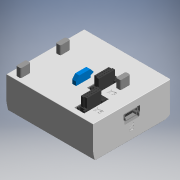
# Autodesk Inventor part: 8070984 CDSB-A1
Saved by Autodesk Inventor 2017.3 (Build 213256000, 256)
## iProperties
Part Number: 8070984 CDSB-A1
Material: Generic
Catalog Web Link: www.cadenas.de
Description: CDSB-Operator unit
Vendor: FESTO
Document SubType Name: Modeling
Designer: partserver
Manufacturer: FESTO
Mass: 36.6 g
Surface Area: 99.6497 cm^2
Volume: 42.8826 cm^3
Density: 1 g/cm^3
Appearance: PSOLRGB-175-175-175
Category: PARTsolutions
Company: FESTO
Title: 8070984 CDSB-A1
Author: Cadenas PARTsolutions
Comments: Operator unit
PSOL_IDENT_0: {$CADENAS_DATA\23d-libs\festo\parts\c\cdsb\cdsb.prj},168 {VTYP=3D},{NB=8070984 CDSB-A1},{LINA=807098
PSOL_IDENT_1: 4 CDSB-A1},{NN=CDSB},{DATE=28.02.2020 14:10:31},{GEOMDATE=22.06.2018 09:50:38},{VERSION=},{LINEID=10
PSOL_IDENT_2: },{WBVAR=},{WBNUMERIC=}  {NB=8070984 CDSB-A1},{LINA=8070984 CDSB-A1},{KT=DUMMY},{TNR=8070984},{TYP=C
PSOL_IDENT_3: DSB-A1},{CNSMASSEXACT=0.0366}
NB: 8070984 CDSB-A1
NN: CDSB
NT: Operator unit
NBSYN: $TNR. $TYP.
LINA: 8070984 CDSB-A1
CATALOG: Festo
TNR: 8070984
TYP: CDSB-A1
CNSMASSEXACT: 0.0366
SUPPLIER: FESTO
ARTICLENO: 8070984 CDSB-A1
BOMINFO: 8070984 CDSB-A1
CREATOR: CADENAS GmbH
Autodesk Inventor part; units mm, degrees
ref_plane "YZ Plane" through (0, 0, 0) normal (1, 0, 0) x (0, 1, 0)
ref_plane "XZ Plane" through (0, 0, 0) normal (0, 1, 0) x (-1, 0, 0)
ref_plane "XY Plane" through (0, 0, 0) normal (0, 0, 1) x (1, 0, 0)
sketch "Sketch_1" plane through (0, 0, 0) normal (1, 0, 0) x (0, 1, 0)
  line L0 (37.9928, 19.588) -> (8.2914, 19.588)
  arc A0 (8.2914, 19.588) -> (1.2796, 18.6197) centre (13.185, -41.717) ccw
  arc A1 (1.2796, 18.6197) -> (1.0492, 18.4076) centre (1.3377, 18.3253) ccw
  arc A2 (1.0492, 18.4076) -> (0, 12.918) centre (31.3426, 9.7728) ccw
  line L1 (0, 12.918) -> (0, 0.2)
  arc A3 (0, 0.2) -> (0.2, 0) centre (0.2, 0.2) ccw
  line L2 (0.2, 0) -> (44.8, 0)
  arc A4 (44.8, 0) -> (45, 0.2) centre (44.8, 0.2) ccw
  line L3 (45, 0.2) -> (45, 17.0653)
  arc A5 (45, 17.0653) -> (44.8438, 17.3286) centre (44.7, 17.0653) ccw
  arc A6 (44.8438, 17.3286) -> (37.9928, 19.588) centre (35.257, -0.224) ccw
  constraints: 14 point on circle, 8 end point, 7 centre point
extrude "Extrusion1" add sketch "Sketch_1" along normal mid plane 50
sketch "Sketch_2" plane through (0, 0, 0) normal (0, 1, 0) x (-1, 0, 0)
  line L0 (30, 25) -> (-30, 25)
  line L1 (-30, 25) -> (-30, -5)
  line L2 (-30, -5) -> (30, -5)
  line L3 (30, -5) -> (30, 25)
  line L4 (25, 0.2) -> (25, 18.5987)
  arc A0 (25, 18.5987) -> (24.7656, 18.8915) centre (24.7, 18.5987) ccw
  arc A1 (24.7656, 18.8915) -> (20, 19.588) centre (17.7679, -12.3341) ccw
  line L5 (20, 19.588) -> (-20, 19.588)
  arc A2 (-20, 19.588) -> (-24.7656, 18.8915) centre (-17.7679, -12.3341) ccw
  arc A3 (-24.7656, 18.8915) -> (-25, 18.5987) centre (-24.7, 18.5987) ccw
  line L6 (-25, 18.5987) -> (-25, 0.2)
  arc A4 (-25, 0.2) -> (-24.8, 0) centre (-24.8, 0.2) ccw
  line L7 (-24.8, 0) -> (24.8, 0)
  arc A5 (24.8, 0) -> (25, 0.2) centre (24.8, 0.2) ccw
  constraints: 16 end point, 12 point on circle, 6 centre point
extrude "Extrusion2" cut sketch "Sketch_2" along normal blind 50
sketch "Sketch_3" plane through (0, 0, 0) normal (0, 0, 1) x (1, 0, 0)
  line L0 (-30, 35) -> (-25, 35)
  line L1 (-25, 35) -> (-25, 44.2)
  arc A0 (-24.2, 45) -> (-25, 44.2) centre (-24.2, 44.2) ccw
  line L2 (-24.2, 45) -> (24.2, 45)
  arc A1 (25, 44.2) -> (24.2, 45) centre (24.2, 44.2) ccw
  line L3 (25, 44.2) -> (25, 35)
  line L4 (25, 35) -> (30, 35)
  line L5 (30, 35) -> (30, 50)
  line L6 (30, 50) -> (-30, 50)
  line L7 (-30, 50) -> (-30, 35)
  constraints: 16 end point, 4 point on circle, 2 centre point
extrude "Extrusion3" cut sketch "Sketch_3" along normal blind 20
sketch "Sketch_4" plane through (0, 0, 0) normal (1, 0, 0) x (0, 1, 0)
  line L0 (45.89, 10.51) -> (45, 10.51)
  line L1 (45, 10.51) -> (45, 2.16)
  line L2 (45, 2.16) -> (45.89, 2.16)
  arc A0 (45.89, 2.16) -> (46.69, 2.96) centre (45.89, 2.96) ccw
  line L3 (46.69, 2.96) -> (46.69, 9.71)
  arc A1 (46.69, 9.71) -> (45.89, 10.51) centre (45.89, 9.71) ccw
  constraints: 8 end point, 4 point on circle, 2 centre point
extrude "Extrusion4" add sketch "Sketch_4" along normal mid plane 21.6
sketch "Sketch_5" plane through (0, 0, 0) normal (0, 0, 1) x (1, 0, 0)
  line L0 (-12.8, 48.69) -> (-12.8, 45)
  line L1 (-12.8, 45) -> (-10.8, 45)
  line L2 (-10.8, 45) -> (-10.8, 46.14)
  arc A0 (-10.25, 46.69) -> (-10.8, 46.14) centre (-10.25, 46.14) ccw
  line L3 (-10.25, 46.69) -> (10.25, 46.69)
  arc A1 (10.8, 46.14) -> (10.25, 46.69) centre (10.25, 46.14) ccw
  line L4 (10.8, 46.14) -> (10.8, 45)
  line L5 (10.8, 45) -> (12.8, 45)
  line L6 (12.8, 45) -> (12.8, 48.69)
  line L7 (12.8, 48.69) -> (-12.8, 48.69)
  constraints: 16 end point, 4 point on circle, 2 centre point
extrude "Extrusion5" cut sketch "Sketch_5" along normal blind 15
sketch "Sketch_6" plane through (0, 0, 0) normal (1, 0, 0) x (0, 1, 0)
  line L0 (22.64, 0) -> (14.2, 0)
  line L1 (14.2, 0) -> (14.2, -2.17)
  line L2 (14.2, -2.17) -> (15.9896, -4.38)
  line L3 (15.9896, -4.38) -> (22.1436, -4.38)
  arc A0 (22.1436, -4.38) -> (22.5649, -4.1835) centre (22.1436, -3.83) ccw
  line L4 (22.5649, -4.1835) -> (24.33, -2.08)
  line L5 (24.33, -2.08) -> (24.33, -1.9851)
  line L6 (24.33, -1.9851) -> (22.64, -1.3364)
  line L7 (22.64, -1.3364) -> (22.64, 0)
  constraints: 16 end point, 2 point on circle, 1 centre point
extrude "Extrusion6" add sketch "Sketch_6" along normal mid plane 2.3
sketch "Sketch_7" plane through (0, 0, 0) normal (0, 0, 1) x (1, 0, 0)
  line L0 (-10.837, 30.43) -> (-10.837, 16.63)
  arc A0 (-10.837, 16.63) -> (-10.637, 16.43) centre (-10.637, 16.63) ccw
  line L1 (-10.637, 16.43) -> (-5.337, 16.43)
  arc A1 (-5.337, 16.43) -> (-5.137, 16.63) centre (-5.337, 16.63) ccw
  line L2 (-5.137, 16.63) -> (-5.137, 30.43)
  arc A2 (-5.137, 30.43) -> (-5.337, 30.63) centre (-5.337, 30.43) ccw
  line L3 (-5.337, 30.63) -> (-10.637, 30.63)
  arc A3 (-10.637, 30.63) -> (-10.837, 30.43) centre (-10.637, 30.43) ccw
  constraints: 8 end point, 8 point on circle, 4 centre point
extrude "Extrusion7" cut sketch "Sketch_7" along normal blind 4.5
sketch "Sketch_8" plane through (0, 0, 0) normal (0, 0, 1) x (1, 0, 0)
  line L0 (-17.136, 16.87) -> (-17.136, 3.07)
  arc A0 (-17.136, 3.07) -> (-16.936, 2.87) centre (-16.936, 3.07) ccw
  line L1 (-16.936, 2.87) -> (-11.636, 2.87)
  arc A1 (-11.636, 2.87) -> (-11.436, 3.07) centre (-11.636, 3.07) ccw
  line L2 (-11.436, 3.07) -> (-11.436, 16.87)
  arc A2 (-11.436, 16.87) -> (-11.636, 17.07) centre (-11.636, 16.87) ccw
  line L3 (-11.636, 17.07) -> (-16.936, 17.07)
  arc A3 (-16.936, 17.07) -> (-17.136, 16.87) centre (-16.936, 16.87) ccw
  constraints: 8 end point, 8 point on circle, 4 centre point
extrude "Extrusion8" cut sketch "Sketch_8" along normal blind 4.5
sketch "Sketch_9" plane through (0, 0, -0.15) normal (0, 0, 1) x (1, 0, 0)
  line L0 (-10.055, 19.535) -> (-10.055, 17.22)
  line L1 (-10.055, 17.22) -> (-9.255, 17.22)
  line L2 (-9.255, 17.22) -> (-9.255, 18.385)
  line L3 (-9.255, 18.385) -> (-6.655, 18.385)
  line L4 (-6.655, 18.385) -> (-6.655, 17.22)
  line L5 (-6.655, 17.22) -> (-5.855, 17.22)
  line L6 (-5.855, 17.22) -> (-5.855, 19.535)
  line L7 (-5.855, 19.535) -> (-6.43, 19.535)
  line L8 (-6.43, 19.535) -> (-6.43, 27.605)
  line L9 (-6.43, 27.605) -> (-5.855, 27.605)
  line L10 (-5.855, 27.605) -> (-5.855, 29.92)
  line L11 (-5.855, 29.92) -> (-6.655, 29.92)
  line L12 (-6.655, 29.92) -> (-6.655, 28.755)
  line L13 (-6.655, 28.755) -> (-9.255, 28.755)
  line L14 (-9.255, 28.755) -> (-9.255, 29.92)
  line L15 (-9.255, 29.92) -> (-10.055, 29.92)
  line L16 (-10.055, 29.92) -> (-10.055, 27.605)
  line L17 (-10.055, 27.605) -> (-9.48, 27.605)
  line L18 (-9.48, 27.605) -> (-9.48, 19.535)
  line L19 (-9.48, 19.535) -> (-10.055, 19.535)
  constraints: 40 end point
extrude "Extrusion9" add sketch "Sketch_9" along normal blind 4.65
sketch "Sketch_10" plane through (0, 0, -0.15) normal (0, 0, 1) x (1, 0, 0)
  line L0 (-16.35, 5.975) -> (-16.35, 3.66)
  line L1 (-16.35, 3.66) -> (-15.55, 3.66)
  line L2 (-15.55, 3.66) -> (-15.55, 4.825)
  line L3 (-15.55, 4.825) -> (-12.95, 4.825)
  line L4 (-12.95, 4.825) -> (-12.95, 3.66)
  line L5 (-12.95, 3.66) -> (-12.15, 3.66)
  line L6 (-12.15, 3.66) -> (-12.15, 5.975)
  line L7 (-12.15, 5.975) -> (-12.725, 5.975)
  line L8 (-12.725, 5.975) -> (-12.725, 14.045)
  line L9 (-12.725, 14.045) -> (-12.15, 14.045)
  line L10 (-12.15, 14.045) -> (-12.15, 16.36)
  line L11 (-12.15, 16.36) -> (-12.95, 16.36)
  line L12 (-12.95, 16.36) -> (-12.95, 15.195)
  line L13 (-12.95, 15.195) -> (-15.55, 15.195)
  line L14 (-15.55, 15.195) -> (-15.55, 16.36)
  line L15 (-15.55, 16.36) -> (-16.35, 16.36)
  line L16 (-16.35, 16.36) -> (-16.35, 14.045)
  line L17 (-16.35, 14.045) -> (-15.775, 14.045)
  line L18 (-15.775, 14.045) -> (-15.775, 5.975)
  line L19 (-15.775, 5.975) -> (-16.35, 5.975)
  constraints: 40 end point
extrude "Extrusion10" add sketch "Sketch_10" along normal blind 4.65
sketch "Sketch_11" plane through (0, 0, -5.35) normal (0, 0, 1) x (1, 0, 0)
  line L0 (-9.48, 18.96) -> (-7.93, 18.96)
  line L1 (-7.93, 18.96) -> (-7.93, 19.46)
  line L2 (-7.93, 19.46) -> (-6.43, 19.46)
  line L3 (-6.43, 19.46) -> (-6.43, 27.83)
  line L4 (-6.43, 27.83) -> (-7.93, 27.83)
  line L5 (-7.93, 27.83) -> (-7.93, 28.33)
  line L6 (-7.93, 28.33) -> (-9.48, 28.33)
  line L7 (-9.48, 28.33) -> (-9.48, 18.96)
  constraints: 16 end point
extrude "Extrusion11" add sketch "Sketch_11" along normal blind 5.2
sketch "Sketch_12" plane through (0, 0, -5.35) normal (0, 0, 1) x (1, 0, 0)
  line L0 (-15.775, 5.83) -> (-14.275, 5.83)
  line L1 (-14.275, 5.83) -> (-14.275, 5.33)
  line L2 (-14.275, 5.33) -> (-12.725, 5.33)
  line L3 (-12.725, 5.33) -> (-12.725, 14.7)
  line L4 (-12.725, 14.7) -> (-14.275, 14.7)
  line L5 (-14.275, 14.7) -> (-14.275, 14.2)
  line L6 (-14.275, 14.2) -> (-15.775, 14.2)
  line L7 (-15.775, 14.2) -> (-15.775, 5.83)
  constraints: 16 end point
extrude "Extrusion12" add sketch "Sketch_12" along normal blind 5.2
sketch "Sketch_13" plane through (0, 0, -5.35) normal (0, 0, 1) x (1, 0, 0)
  line L0 (-8.7, 26.53) -> (-8.3, 26.53)
  line L1 (-8.3, 26.53) -> (-8.3, 27.13)
  line L2 (-8.3, 27.13) -> (-8.7, 27.13)
  line L3 (-8.7, 27.13) -> (-8.7, 26.53)
  constraints: 8 end point
extrude "Extrusion13" cut sketch "Sketch_13" along normal blind 0.5
sketch "Pattern_1_SKETCH_1" plane through (0, 0, -5.35) normal (0, 0, 1) x (1, 0, 0)
  line L0 (-7.43, 26.53) -> (-7.03, 26.53)
  line L1 (-7.03, 26.53) -> (-7.03, 27.13)
  line L2 (-7.03, 27.13) -> (-7.43, 27.13)
  line L3 (-7.43, 27.13) -> (-7.43, 26.53)
  constraints: 8 end point
sketch "Pattern_1_SKETCH_2" plane through (0, 0, -5.35) normal (0, 0, 1) x (1, 0, 0)
  line L0 (-7.43, 25.26) -> (-7.03, 25.26)
  line L1 (-7.03, 25.26) -> (-7.03, 25.86)
  line L2 (-7.03, 25.86) -> (-7.43, 25.86)
  line L3 (-7.43, 25.86) -> (-7.43, 25.26)
  constraints: 8 end point
sketch "Pattern_1_SKETCH_3" plane through (0, 0, -5.35) normal (0, 0, 1) x (1, 0, 0)
  line L0 (-7.43, 23.99) -> (-7.03, 23.99)
  line L1 (-7.03, 23.99) -> (-7.03, 24.59)
  line L2 (-7.03, 24.59) -> (-7.43, 24.59)
  line L3 (-7.43, 24.59) -> (-7.43, 23.99)
  constraints: 8 end point
sketch "Pattern_1_SKETCH_4" plane through (0, 0, -5.35) normal (0, 0, 1) x (1, 0, 0)
  line L0 (-7.43, 22.72) -> (-7.03, 22.72)
  line L1 (-7.03, 22.72) -> (-7.03, 23.32)
  line L2 (-7.03, 23.32) -> (-7.43, 23.32)
  line L3 (-7.43, 23.32) -> (-7.43, 22.72)
  constraints: 8 end point
sketch "Pattern_1_SKETCH_5" plane through (0, 0, -5.35) normal (0, 0, 1) x (1, 0, 0)
  line L0 (-7.43, 21.45) -> (-7.03, 21.45)
  line L1 (-7.03, 21.45) -> (-7.03, 22.05)
  line L2 (-7.03, 22.05) -> (-7.43, 22.05)
  line L3 (-7.43, 22.05) -> (-7.43, 21.45)
  constraints: 8 end point
sketch "Pattern_1_SKETCH_6" plane through (0, 0, -5.35) normal (0, 0, 1) x (1, 0, 0)
  line L0 (-7.43, 20.18) -> (-7.03, 20.18)
  line L1 (-7.03, 20.18) -> (-7.03, 20.78)
  line L2 (-7.03, 20.78) -> (-7.43, 20.78)
  line L3 (-7.43, 20.78) -> (-7.43, 20.18)
  constraints: 8 end point
sketch "Pattern_1_SKETCH_7" plane through (0, 0, -5.35) normal (0, 0, 1) x (1, 0, 0)
  line L0 (-8.7, 25.26) -> (-8.3, 25.26)
  line L1 (-8.3, 25.26) -> (-8.3, 25.86)
  line L2 (-8.3, 25.86) -> (-8.7, 25.86)
  line L3 (-8.7, 25.86) -> (-8.7, 25.26)
  constraints: 8 end point
sketch "Pattern_1_SKETCH_8" plane through (0, 0, -5.35) normal (0, 0, 1) x (1, 0, 0)
  line L0 (-8.7, 23.99) -> (-8.3, 23.99)
  line L1 (-8.3, 23.99) -> (-8.3, 24.59)
  line L2 (-8.3, 24.59) -> (-8.7, 24.59)
  line L3 (-8.7, 24.59) -> (-8.7, 23.99)
  constraints: 8 end point
sketch "Pattern_1_SKETCH_9" plane through (0, 0, -5.35) normal (0, 0, 1) x (1, 0, 0)
  line L0 (-8.7, 22.72) -> (-8.3, 22.72)
  line L1 (-8.3, 22.72) -> (-8.3, 23.32)
  line L2 (-8.3, 23.32) -> (-8.7, 23.32)
  line L3 (-8.7, 23.32) -> (-8.7, 22.72)
  constraints: 8 end point
sketch "Pattern_1_SKETCH_10" plane through (0, 0, -5.35) normal (0, 0, 1) x (1, 0, 0)
  line L0 (-8.7, 21.45) -> (-8.3, 21.45)
  line L1 (-8.3, 21.45) -> (-8.3, 22.05)
  line L2 (-8.3, 22.05) -> (-8.7, 22.05)
  line L3 (-8.7, 22.05) -> (-8.7, 21.45)
  constraints: 8 end point
sketch "Pattern_1_SKETCH_11" plane through (0, 0, -5.35) normal (0, 0, 1) x (1, 0, 0)
  line L0 (-8.7, 20.18) -> (-8.3, 20.18)
  line L1 (-8.3, 20.18) -> (-8.3, 20.78)
  line L2 (-8.3, 20.78) -> (-8.7, 20.78)
  line L3 (-8.7, 20.78) -> (-8.7, 20.18)
  constraints: 8 end point
sketch "Pattern_1_SKETCH_12" plane through (0, 0, -5.35) normal (0, 0, 1) x (1, 0, 0)
  line L0 (-15, 12.97) -> (-14.6, 12.97)
  line L1 (-14.6, 12.97) -> (-14.6, 13.57)
  line L2 (-14.6, 13.57) -> (-15, 13.57)
  line L3 (-15, 13.57) -> (-15, 12.97)
  constraints: 8 end point
sketch "Pattern_1_SKETCH_13" plane through (0, 0, -5.35) normal (0, 0, 1) x (1, 0, 0)
  line L0 (-13.73, 12.97) -> (-13.33, 12.97)
  line L1 (-13.33, 12.97) -> (-13.33, 13.57)
  line L2 (-13.33, 13.57) -> (-13.73, 13.57)
  line L3 (-13.73, 13.57) -> (-13.73, 12.97)
  constraints: 8 end point
sketch "Pattern_1_SKETCH_14" plane through (0, 0, -5.35) normal (0, 0, 1) x (1, 0, 0)
  line L0 (-15, 11.7) -> (-14.6, 11.7)
  line L1 (-14.6, 11.7) -> (-14.6, 12.3)
  line L2 (-14.6, 12.3) -> (-15, 12.3)
  line L3 (-15, 12.3) -> (-15, 11.7)
  constraints: 8 end point
sketch "Pattern_1_SKETCH_15" plane through (0, 0, -5.35) normal (0, 0, 1) x (1, 0, 0)
  line L0 (-13.73, 11.7) -> (-13.33, 11.7)
  line L1 (-13.33, 11.7) -> (-13.33, 12.3)
  line L2 (-13.33, 12.3) -> (-13.73, 12.3)
  line L3 (-13.73, 12.3) -> (-13.73, 11.7)
  constraints: 8 end point
sketch "Pattern_1_SKETCH_16" plane through (0, 0, -5.35) normal (0, 0, 1) x (1, 0, 0)
  line L0 (-15, 10.43) -> (-14.6, 10.43)
  line L1 (-14.6, 10.43) -> (-14.6, 11.03)
  line L2 (-14.6, 11.03) -> (-15, 11.03)
  line L3 (-15, 11.03) -> (-15, 10.43)
  constraints: 8 end point
sketch "Pattern_1_SKETCH_17" plane through (0, 0, -5.35) normal (0, 0, 1) x (1, 0, 0)
  line L0 (-13.73, 10.43) -> (-13.33, 10.43)
  line L1 (-13.33, 10.43) -> (-13.33, 11.03)
  line L2 (-13.33, 11.03) -> (-13.73, 11.03)
  line L3 (-13.73, 11.03) -> (-13.73, 10.43)
  constraints: 8 end point
sketch "Pattern_1_SKETCH_18" plane through (0, 0, -5.35) normal (0, 0, 1) x (1, 0, 0)
  line L0 (-15, 9.16) -> (-14.6, 9.16)
  line L1 (-14.6, 9.16) -> (-14.6, 9.76)
  line L2 (-14.6, 9.76) -> (-15, 9.76)
  line L3 (-15, 9.76) -> (-15, 9.16)
  constraints: 8 end point
sketch "Pattern_1_SKETCH_19" plane through (0, 0, -5.35) normal (0, 0, 1) x (1, 0, 0)
  line L0 (-13.73, 9.16) -> (-13.33, 9.16)
  line L1 (-13.33, 9.16) -> (-13.33, 9.76)
  line L2 (-13.33, 9.76) -> (-13.73, 9.76)
  line L3 (-13.73, 9.76) -> (-13.73, 9.16)
  constraints: 8 end point
sketch "Pattern_1_SKETCH_20" plane through (0, 0, -5.35) normal (0, 0, 1) x (1, 0, 0)
  line L0 (-15, 7.89) -> (-14.6, 7.89)
  line L1 (-14.6, 7.89) -> (-14.6, 8.49)
  line L2 (-14.6, 8.49) -> (-15, 8.49)
  line L3 (-15, 8.49) -> (-15, 7.89)
  constraints: 8 end point
sketch "Pattern_1_SKETCH_21" plane through (0, 0, -5.35) normal (0, 0, 1) x (1, 0, 0)
  line L0 (-13.73, 7.89) -> (-13.33, 7.89)
  line L1 (-13.33, 7.89) -> (-13.33, 8.49)
  line L2 (-13.33, 8.49) -> (-13.73, 8.49)
  line L3 (-13.73, 8.49) -> (-13.73, 7.89)
  constraints: 8 end point
sketch "Pattern_1_SKETCH_22" plane through (0, 0, -5.35) normal (0, 0, 1) x (1, 0, 0)
  line L0 (-15, 6.62) -> (-14.6, 6.62)
  line L1 (-14.6, 6.62) -> (-14.6, 7.22)
  line L2 (-14.6, 7.22) -> (-15, 7.22)
  line L3 (-15, 7.22) -> (-15, 6.62)
  constraints: 8 end point
sketch "Pattern_1_SKETCH_23" plane through (0, 0, -5.35) normal (0, 0, 1) x (1, 0, 0)
  line L0 (-13.73, 6.62) -> (-13.33, 6.62)
  line L1 (-13.33, 6.62) -> (-13.33, 7.22)
  line L2 (-13.33, 7.22) -> (-13.73, 7.22)
  line L3 (-13.73, 7.22) -> (-13.73, 6.62)
  constraints: 8 end point
extrude "Extrusion14" cut sketch "Pattern_1_SKETCH_1" along normal blind 0.5
extrude "Extrusion15" cut sketch "Pattern_1_SKETCH_2" along normal blind 0.5
extrude "Extrusion16" cut sketch "Pattern_1_SKETCH_3" along normal blind 0.5
extrude "Extrusion17" cut sketch "Pattern_1_SKETCH_4" along normal blind 0.5
extrude "Extrusion18" cut sketch "Pattern_1_SKETCH_5" along normal blind 0.5
extrude "Extrusion19" cut sketch "Pattern_1_SKETCH_6" along normal blind 0.5
extrude "Extrusion20" cut sketch "Pattern_1_SKETCH_7" along normal blind 0.5
extrude "Extrusion21" cut sketch "Pattern_1_SKETCH_8" along normal blind 0.5
extrude "Extrusion22" cut sketch "Pattern_1_SKETCH_9" along normal blind 0.5
extrude "Extrusion23" cut sketch "Pattern_1_SKETCH_10" along normal blind 0.5
extrude "Extrusion24" cut sketch "Pattern_1_SKETCH_11" along normal blind 0.5
extrude "Extrusion25" cut sketch "Pattern_1_SKETCH_12" along normal blind 0.5
extrude "Extrusion26" cut sketch "Pattern_1_SKETCH_13" along normal blind 0.5
extrude "Extrusion27" cut sketch "Pattern_1_SKETCH_14" along normal blind 0.5
extrude "Extrusion28" cut sketch "Pattern_1_SKETCH_15" along normal blind 0.5
extrude "Extrusion29" cut sketch "Pattern_1_SKETCH_16" along normal blind 0.5
extrude "Extrusion30" cut sketch "Pattern_1_SKETCH_17" along normal blind 0.5
extrude "Extrusion31" cut sketch "Pattern_1_SKETCH_18" along normal blind 0.5
extrude "Extrusion32" cut sketch "Pattern_1_SKETCH_19" along normal blind 0.5
extrude "Extrusion33" cut sketch "Pattern_1_SKETCH_20" along normal blind 0.5
extrude "Extrusion34" cut sketch "Pattern_1_SKETCH_21" along normal blind 0.5
extrude "Extrusion35" cut sketch "Pattern_1_SKETCH_22" along normal blind 0.5
extrude "Extrusion36" cut sketch "Pattern_1_SKETCH_23" along normal blind 0.5
sketch "Sketch_15" plane through (0, 0, 0) normal (0, 0, 1) x (1, 0, 0)
  arc A0 (18.65, 25.55) -> (19.35, 24.85) centre (19.35, 25.55) ccw
  line L0 (19.35, 24.85) -> (20.7, 24.85)
  arc A1 (20.7, 24.85) -> (21.4, 25.55) centre (20.7, 25.55) ccw
  line L1 (21.4, 25.55) -> (21.4, 29.9)
  arc A2 (21.4, 29.9) -> (20.7, 30.6) centre (20.7, 29.9) ccw
  line L2 (20.7, 30.6) -> (19.35, 30.6)
  arc A3 (19.35, 30.6) -> (18.65, 29.9) centre (19.35, 29.9) ccw
  line L3 (18.65, 29.9) -> (18.65, 25.55)
  constraints: 8 end point, 8 point on circle, 4 centre point
extrude "Extrusion37" add sketch "Sketch_15" against normal blind 5
sketch "Sketch_16" plane through (0, 0, 0) normal (0, 0, 1) x (1, 0, 0)
  arc A0 (18.65, 2.7) -> (19.35, 2) centre (19.35, 2.7) ccw
  line L0 (19.35, 2) -> (20.7, 2)
  arc A1 (20.7, 2) -> (21.4, 2.7) centre (20.7, 2.7) ccw
  line L1 (21.4, 2.7) -> (21.4, 7.05)
  arc A2 (21.4, 7.05) -> (20.7, 7.75) centre (20.7, 7.05) ccw
  line L2 (20.7, 7.75) -> (19.35, 7.75)
  arc A3 (19.35, 7.75) -> (18.65, 7.05) centre (19.35, 7.05) ccw
  line L3 (18.65, 7.05) -> (18.65, 2.7)
  constraints: 8 end point, 8 point on circle, 4 centre point
extrude "Extrusion38" add sketch "Sketch_16" against normal blind 5
sketch "Sketch_17" plane through (0, 0, 0) normal (0, 0, 1) x (1, 0, 0)
  arc A0 (-16.1, 25.55) -> (-15.4, 24.85) centre (-15.4, 25.55) ccw
  line L0 (-15.4, 24.85) -> (-14.05, 24.85)
  arc A1 (-14.05, 24.85) -> (-13.35, 25.55) centre (-14.05, 25.55) ccw
  line L1 (-13.35, 25.55) -> (-13.35, 29.9)
  arc A2 (-13.35, 29.9) -> (-14.05, 30.6) centre (-14.05, 29.9) ccw
  line L2 (-14.05, 30.6) -> (-15.4, 30.6)
  arc A3 (-15.4, 30.6) -> (-16.1, 29.9) centre (-15.4, 29.9) ccw
  line L3 (-16.1, 29.9) -> (-16.1, 25.55)
  constraints: 8 end point, 8 point on circle, 4 centre point
extrude "Extrusion39" add sketch "Sketch_17" against normal blind 5
sketch "Sketch_18" plane through (-18.6, 0, 0) normal (1, 0, 0) x (0, 0, -1)
  line L0 (-9.6, 26.25) -> (-9.6, 18.75)
  arc A0 (-9.6, 18.75) -> (-9.1, 18.25) centre (-9.1, 18.75) ccw
  line L1 (-9.1, 18.25) -> (-8.1203, 18.25)
  arc A1 (-7.8972, 18.1975) -> (-8.1203, 18.25) centre (-8.1203, 17.75) ccw
  line L2 (-7.8972, 18.1975) -> (-7.1051, 17.8025)
  arc A2 (-7.1051, 17.8025) -> (-6.882, 17.75) centre (-6.882, 18.25) ccw
  line L3 (-6.882, 17.75) -> (-4.5, 17.75)
  arc A3 (-4.5, 17.75) -> (-4, 18.25) centre (-4.5, 18.25) ccw
  line L4 (-4, 18.25) -> (-4, 26.75)
  arc A4 (-4, 26.75) -> (-4.5, 27.25) centre (-4.5, 26.75) ccw
  line L5 (-4.5, 27.25) -> (-6.882, 27.25)
  arc A5 (-6.882, 27.25) -> (-7.1051, 27.1975) centre (-6.882, 26.75) ccw
  line L6 (-7.1051, 27.1975) -> (-7.8972, 26.8025)
  arc A6 (-8.1203, 26.75) -> (-7.8972, 26.8025) centre (-8.1203, 27.25) ccw
  line L7 (-8.1203, 26.75) -> (-9.1, 26.75)
  arc A7 (-9.1, 26.75) -> (-9.6, 26.25) centre (-9.1, 26.25) ccw
  constraints: 16 end point, 16 point on circle, 8 centre point
extrude "Extrusion40" cut sketch "Sketch_18" against normal blind 6.5
sketch "Sketch_19" plane through (-18.6, 0, 0) normal (1, 0, 0) x (0, 0, -1)
  line L0 (-8.6, 25.335) -> (-8.6, 19.665)
  arc A0 (-8.6, 19.665) -> (-8.1, 19.165) centre (-8.1, 19.665) ccw
  line L1 (-8.1, 19.165) -> (-7.354, 19.165)
  arc A1 (-7.2986, 19.1482) -> (-7.354, 19.165) centre (-7.354, 19.065) ccw
  line L2 (-7.2986, 19.1482) -> (-6.6775, 18.734)
  arc A2 (-6.6775, 18.734) -> (-6.4001, 18.65) centre (-6.4001, 19.15) ccw
  line L3 (-6.4001, 18.65) -> (-5.2, 18.65)
  arc A3 (-5.2, 18.65) -> (-4.7, 19.15) centre (-5.2, 19.15) ccw
  line L4 (-4.7, 19.15) -> (-4.7, 25.85)
  arc A4 (-4.7, 25.85) -> (-5.2, 26.35) centre (-5.2, 25.85) ccw
  line L5 (-5.2, 26.35) -> (-6.4001, 26.35)
  arc A5 (-6.4001, 26.35) -> (-6.6775, 26.266) centre (-6.4001, 25.85) ccw
  line L6 (-6.6775, 26.266) -> (-7.2986, 25.8518)
  arc A6 (-7.354, 25.835) -> (-7.2986, 25.8518) centre (-7.354, 25.935) ccw
  line L7 (-7.354, 25.835) -> (-8.1, 25.835)
  arc A7 (-8.1, 25.835) -> (-8.6, 25.335) centre (-8.1, 25.335) ccw
  line L8 (-8.2, 25.335) -> (-8.2, 19.665)
  arc A8 (-8.2, 19.665) -> (-8.1, 19.565) centre (-8.1, 19.665) ccw
  line L9 (-8.1, 19.565) -> (-7.354, 19.565)
  arc A9 (-7.0766, 19.481) -> (-7.354, 19.565) centre (-7.354, 19.065) ccw
  line L10 (-7.0766, 19.481) -> (-6.4556, 19.0668)
  arc A10 (-6.4556, 19.0668) -> (-6.4001, 19.05) centre (-6.4001, 19.15) ccw
  line L11 (-6.4001, 19.05) -> (-5.2, 19.05)
  arc A11 (-5.2, 19.05) -> (-5.1, 19.15) centre (-5.2, 19.15) ccw
  line L12 (-5.1, 19.15) -> (-5.1, 25.85)
  arc A12 (-5.1, 25.85) -> (-5.2, 25.95) centre (-5.2, 25.85) ccw
  line L13 (-5.2, 25.95) -> (-6.4001, 25.95)
  arc A13 (-6.4001, 25.95) -> (-6.4556, 25.9332) centre (-6.4001, 25.85) ccw
  line L14 (-6.4556, 25.9332) -> (-7.0766, 25.519)
  arc A14 (-7.354, 25.435) -> (-7.0766, 25.519) centre (-7.354, 25.935) ccw
  line L15 (-7.354, 25.435) -> (-8.1, 25.435)
  arc A15 (-8.1, 25.435) -> (-8.2, 25.335) centre (-8.1, 25.335) ccw
  constraints: 32 end point, 32 point on circle, 16 centre point
extrude "Extrusion41" add sketch "Sketch_19" against normal blind 5.9
sketch "Sketch_20" plane through (-18.6, 0, 0) normal (1, 0, 0) x (0, 0, -1)
  arc A0 (-7.63, 20.5388) -> (-7.5609, 20.4437) centre (-7.53, 20.5388) ccw
  line L0 (-7.5609, 20.4437) -> (-6.8874, 20.2249)
  arc A1 (-6.8874, 20.2249) -> (-6.8565, 20.22) centre (-6.8565, 20.32) ccw
  line L1 (-6.8565, 20.22) -> (-6.15, 20.22)
  arc A2 (-6.15, 20.22) -> (-6.05, 20.32) centre (-6.15, 20.32) ccw
  line L2 (-6.05, 20.32) -> (-6.05, 24.67)
  arc A3 (-6.05, 24.67) -> (-6.15, 24.77) centre (-6.15, 24.67) ccw
  line L3 (-6.15, 24.77) -> (-6.8565, 24.77)
  arc A4 (-6.8565, 24.77) -> (-6.8874, 24.7651) centre (-6.8565, 24.67) ccw
  line L4 (-6.8874, 24.7651) -> (-7.5609, 24.5463)
  arc A5 (-7.5609, 24.5463) -> (-7.63, 24.4512) centre (-7.53, 24.4512) ccw
  line L5 (-7.63, 24.4512) -> (-7.63, 20.5388)
  line L6 (-6.87, 23.895) -> (-6.3, 23.895)
  line L7 (-6.3, 23.895) -> (-6.3, 24.295)
  line L8 (-6.3, 24.295) -> (-6.87, 24.295)
  line L9 (-6.87, 24.295) -> (-6.87, 23.895)
  line L10 (-6.87, 23.095) -> (-6.3, 23.095)
  line L11 (-6.3, 23.095) -> (-6.3, 23.495)
  line L12 (-6.3, 23.495) -> (-6.87, 23.495)
  line L13 (-6.87, 23.495) -> (-6.87, 23.095)
  line L14 (-6.87, 22.295) -> (-6.3, 22.295)
  line L15 (-6.3, 22.295) -> (-6.3, 22.695)
  line L16 (-6.3, 22.695) -> (-6.87, 22.695)
  line L17 (-6.87, 22.695) -> (-6.87, 22.295)
  line L18 (-6.87, 21.495) -> (-6.3, 21.495)
  line L19 (-6.3, 21.495) -> (-6.3, 21.895)
  line L20 (-6.3, 21.895) -> (-6.87, 21.895)
  line L21 (-6.87, 21.895) -> (-6.87, 21.495)
  line L22 (-6.87, 20.695) -> (-6.3, 20.695)
  line L23 (-6.3, 20.695) -> (-6.3, 21.095)
  line L24 (-6.3, 21.095) -> (-6.87, 21.095)
  line L25 (-6.87, 21.095) -> (-6.87, 20.695)
  constraints: 52 end point, 12 point on circle, 6 centre point
extrude "Extrusion42" add sketch "Sketch_20" against normal blind 4.55
sketch "Sketch_21" plane through (0, 0, 19.588) normal (0, 0, 1) x (1, 0, 0)
  line L0 (-20.5, 36.85) -> (-20.5, 8.85)
  arc A0 (-20.5, 8.85) -> (-19.5, 7.85) centre (-19.5, 8.85) ccw
  line L1 (-19.5, 7.85) -> (19.5, 7.85)
  arc A1 (19.5, 7.85) -> (20.5, 8.85) centre (19.5, 8.85) ccw
  line L2 (20.5, 8.85) -> (20.5, 36.85)
  arc A2 (20.5, 36.85) -> (19.5, 37.85) centre (19.5, 36.85) ccw
  line L3 (19.5, 37.85) -> (-19.5, 37.85)
  arc A3 (-19.5, 37.85) -> (-20.5, 36.85) centre (-19.5, 36.85) ccw
  constraints: 8 end point, 8 point on circle, 4 centre point
extrude "Extrusion43" cut sketch "Sketch_21" against normal blind 0.6
sketch "Sketch_28" plane through (0, 0, 18.988) normal (0, 0, 1) x (1, 0, 0)
  line L0 (-20.5, 36.85) -> (-20.5, 8.85)
  arc A0 (-20.5, 8.85) -> (-19.5, 7.85) centre (-19.5, 8.85) ccw
  line L1 (-19.5, 7.85) -> (-15.5, 7.85)
  line L2 (-15.5, 7.85) -> (-15.5, 37.85)
  line L3 (-15.5, 37.85) -> (-19.5, 37.85)
  arc A1 (-19.5, 37.85) -> (-20.5, 36.85) centre (-19.5, 36.85) ccw
  constraints: 8 end point, 4 point on circle, 2 centre point
extrude "Extrusion44" add sketch "Sketch_28" along normal blind 0.4
sketch "Sketch_22" plane through (-25, 0, 0) normal (1, 0, 0) x (0, 0, -1)
  line L0 (-13.0625, 21.25) -> (-12.6562, 21.25)
  line L1 (-12.6562, 21.25) -> (-12, 22.2188)
  line L2 (-12, 22.2188) -> (-11.3438, 21.25)
  line L3 (-11.3438, 21.25) -> (-10.9375, 21.25)
  line L4 (-10.9375, 21.25) -> (-11.8125, 22.5313)
  line L5 (-11.8125, 22.5313) -> (-10.9688, 23.75)
  line L6 (-10.9688, 23.75) -> (-11.375, 23.75)
  line L7 (-11.375, 23.75) -> (-12, 22.8125)
  line L8 (-12, 22.8125) -> (-12.625, 23.75)
  line L9 (-12.625, 23.75) -> (-13.0312, 23.75)
  line L10 (-13.0312, 23.75) -> (-12.1875, 22.5313)
  line L11 (-12.1875, 22.5313) -> (-13.0625, 21.25)
  constraints: 24 end point
extrude "Extrusion45" cut sketch "Sketch_22" along normal blind 0.3
sketch "Sketch_23" plane through (-25, 0, 0) normal (1, 0, 0) x (0, 0, -1)
  line L0 (-14.5, 21.6) -> (-14.5, 21.25)
  line L1 (-14.5, 21.25) -> (-13.5, 21.25)
  line L2 (-13.5, 21.25) -> (-13.5, 21.6)
  line L3 (-13.5, 21.6) -> (-13.825, 21.6)
  line L4 (-13.825, 21.6) -> (-13.825, 23.25)
  line L5 (-13.825, 23.25) -> (-13.5, 22.75)
  line L6 (-13.5, 22.75) -> (-13.5, 23.25)
  line L7 (-13.5, 23.25) -> (-13.825, 23.75)
  line L8 (-13.825, 23.75) -> (-14.175, 23.75)
  line L9 (-14.175, 23.75) -> (-14.175, 21.6)
  line L10 (-14.175, 21.6) -> (-14.5, 21.6)
  constraints: 22 end point
extrude "Extrusion46" cut sketch "Sketch_23" along normal blind 0.3
sketch "Sketch_25" plane through (0, 0, 0) normal (0, 0, 1) x (1, 0, 0)
  line L0 (-15.0625, 20) -> (-14.6563, 20)
  line L1 (-14.6563, 20) -> (-14, 20.9688)
  line L2 (-14, 20.9688) -> (-13.3438, 20)
  line L3 (-13.3438, 20) -> (-12.9375, 20)
  line L4 (-12.9375, 20) -> (-13.8125, 21.2813)
  line L5 (-13.8125, 21.2813) -> (-12.9688, 22.5)
  line L6 (-12.9688, 22.5) -> (-13.375, 22.5)
  line L7 (-13.375, 22.5) -> (-14, 21.5625)
  line L8 (-14, 21.5625) -> (-14.625, 22.5)
  line L9 (-14.625, 22.5) -> (-15.0312, 22.5)
  line L10 (-15.0312, 22.5) -> (-14.1875, 21.2813)
  line L11 (-14.1875, 21.2813) -> (-15.0625, 20)
  constraints: 24 end point
extrude "Extrusion47" cut sketch "Sketch_25" along normal blind 0.3
sketch "Sketch_24" plane through (0, 0, 0) normal (0, 0, 1) x (1, 0, 0)
  line L0 (-20.0625, 7) -> (-19.6562, 7)
  line L1 (-19.6562, 7) -> (-19, 7.9688)
  line L2 (-19, 7.9688) -> (-18.3438, 7)
  line L3 (-18.3438, 7) -> (-17.9375, 7)
  line L4 (-17.9375, 7) -> (-18.8125, 8.2812)
  line L5 (-18.8125, 8.2812) -> (-17.9688, 9.5)
  line L6 (-17.9688, 9.5) -> (-18.375, 9.5)
  line L7 (-18.375, 9.5) -> (-19, 8.5625)
  line L8 (-19, 8.5625) -> (-19.625, 9.5)
  line L9 (-19.625, 9.5) -> (-20.0313, 9.5)
  line L10 (-20.0313, 9.5) -> (-19.1875, 8.2812)
  line L11 (-19.1875, 8.2812) -> (-20.0625, 7)
  constraints: 24 end point
extrude "Extrusion48" cut sketch "Sketch_24" along normal blind 0.3
sketch "Sketch_26" plane through (0, 0, 0) normal (0, 0, 1) x (1, 0, 0)
  arc A0 (-16.0847, 21.0048) -> (-16.6682, 21.4095) centre (-16, 21.75) ccw
  line L0 (-16.6682, 21.4095) -> (-15.95, 20)
  line L1 (-15.95, 20) -> (-15.6, 20)
  line L2 (-15.6, 20) -> (-16.0847, 21.0048)
  circle A1 centre (-16, 21.75) radius 0.4
  constraints: 6 end point, 2 centre point, 2 point on circle
extrude "Extrusion49" cut sketch "Sketch_26" along normal blind 0.3
sketch "Sketch_27" plane through (0, 0, 0) normal (0, 0, 1) x (1, 0, 0)
  arc A0 (-20.6581, 8.6805) -> (-20.2188, 7.4809) centre (-21, 7.875) ccw
  line L0 (-20.2188, 7.4809) -> (-20.5316, 7.7)
  arc A1 (-20.6429, 8.225) -> (-20.5316, 7.7) centre (-21, 7.875) ccw
  line L1 (-20.6429, 8.225) -> (-20.5457, 8.225)
  line L2 (-20.5457, 8.225) -> (-20.2149, 8.3454)
  line L3 (-20.2149, 8.3454) -> (-20.5, 9.5)
  line L4 (-20.5, 9.5) -> (-21.75, 9.5)
  line L5 (-21.75, 9.5) -> (-21.75, 9.15)
  line L6 (-21.75, 9.15) -> (-20.7741, 9.15)
  line L7 (-20.7741, 9.15) -> (-20.6581, 8.6805)
  constraints: 16 end point, 4 point on circle, 2 centre point
extrude "Extrusion50" cut sketch "Sketch_27" along normal blind 0.3
ref_plane "ANBAU_XY" through (0.06, 22.3, 0) normal (0, 0, -1) x (1, 0, 0)
ref_plane "ANBAU_YZ" through (0.06, 22.3, 0) normal (1, 0, 0) x (0, -1, 0)
ref_plane "ANBAU_ZX" through (0.06, 22.3, 0) normal (0, -1, 0) x (0, 0, -1)
body "Solid1"
